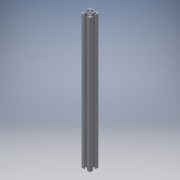
# Autodesk Inventor part: 20-2020_300mm
Saved by Autodesk Inventor 2019.4 (Build 234330000, 330)
## iProperties
Created: 2014-04-23
Part Number: 20-2020_300mm
Material: Aluminum 6105 T-5
Document SubType Name: Modeling
Designer: Ross Bowman
Density: 2.71 g/cm^3
Engineer: Ross Bowman
Catalog Web Link: 8020.net
Vendor: 80/20 Inc.
Mass: 43.1913 g
Surface Area: 184.633 cm^2
Volume: 15.9377 cm^3
Appearance: Aluminum - Flat
Company: 80/20 Inc.
Material: 6105-T5 Aluminum
Author: Ross Bowman
Keywords: 80/20 , 8020 , T-Slot , Extrusion
Autodesk Inventor part; units mm, degrees
ref_plane "YZ Plane" through (0, 0, 0) normal (1, 0, 0) x (0, 1, 0)
ref_plane "XZ Plane" through (0, 0, 0) normal (0, 1, 0) x (-1, 0, 0)
ref_plane "XY Plane" through (0, 0, 0) normal (0, 0, 1) x (1, 0, 0)
sketch "Sketch1" plane through (0, 0, 0) normal (0, 0, 1) x (1, 0, 0)
  arc A0 (-2.1249, -2.3045) -> (-0.804, -1.9351) centre (-1.5684, -1.748) ccw
  line L0 (-2.3045, -2.1249) -> (-2.1249, -2.3045)
  arc A1 (-1.9351, -0.804) -> (-2.3045, -2.1249) centre (-1.748, -1.5684) ccw
  arc A2 (-1.9351, 0.804) -> (-1.9351, -0.804) centre (0, 0) ccw
  arc A3 (-2.3045, 2.1249) -> (-1.9351, 0.804) centre (-1.748, 1.5684) ccw
  line L1 (-2.1249, 2.3045) -> (-2.3045, 2.1249)
  arc A4 (-0.804, 1.9351) -> (-2.1249, 2.3045) centre (-1.5684, 1.748) ccw
  arc A5 (0.804, 1.9351) -> (-0.804, 1.9351) centre (0, 0) ccw
  arc A6 (2.1249, 2.3045) -> (0.804, 1.9351) centre (1.5684, 1.748) ccw
  line L2 (2.3045, 2.1249) -> (2.1249, 2.3045)
  arc A7 (1.9351, 0.804) -> (2.3045, 2.1249) centre (1.748, 1.5684) ccw
  arc A8 (1.9351, -0.804) -> (1.9351, 0.804) centre (0, 0) ccw
  arc A9 (2.3045, -2.1249) -> (1.9351, -0.804) centre (1.748, -1.5684) ccw
  line L3 (2.1249, -2.3045) -> (2.3045, -2.1249)
  arc A10 (0.804, -1.9351) -> (2.1249, -2.3045) centre (1.5684, -1.748) ccw
  arc A11 (-0.804, -1.9351) -> (0.804, -1.9351) centre (0, 0) ccw
  arc A12 (9.492, 2.63) -> (10, 3.138) centre (9.492, 3.138) ccw
  line L4 (10, 3.138) -> (10, 8.5)
  arc A13 (10, 8.5) -> (8.5, 10) centre (8.5, 8.5) ccw
  line L5 (8.5, 10) -> (3.138, 10)
  arc A14 (3.138, 10) -> (2.63, 9.492) centre (3.138, 9.492) ccw
  line L6 (2.63, 9.492) -> (2.63, 9.008)
  arc A15 (2.63, 9.008) -> (3.138, 8.5) centre (3.138, 9.008) ccw
  line L7 (3.138, 8.5) -> (5.487, 8.5)
  arc A16 (5.995, 7.992) -> (5.487, 8.5) centre (5.487, 7.992) ccw
  line L8 (5.995, 7.992) -> (5.995, 7.2661)
  arc A17 (5.8462, 6.9069) -> (5.995, 7.2661) centre (5.487, 7.2661) ccw
  line L9 (5.8462, 6.9069) -> (2.7431, 3.8038)
  arc A18 (2.3839, 3.655) -> (2.7431, 3.8038) centre (2.3839, 4.163) ccw
  line L10 (2.3839, 3.655) -> (-2.3839, 3.655)
  arc A19 (-2.7431, 3.8038) -> (-2.3839, 3.655) centre (-2.3839, 4.163) ccw
  line L11 (-2.7431, 3.8038) -> (-5.8462, 6.9069)
  arc A20 (-5.995, 7.2661) -> (-5.8462, 6.9069) centre (-5.487, 7.2661) ccw
  line L12 (-5.995, 7.2661) -> (-5.995, 7.992)
  arc A21 (-5.487, 8.5) -> (-5.995, 7.992) centre (-5.487, 7.992) ccw
  line L13 (-5.487, 8.5) -> (-3.138, 8.5)
  arc A22 (-3.138, 8.5) -> (-2.63, 9.008) centre (-3.138, 9.008) ccw
  line L14 (-2.63, 9.008) -> (-2.63, 9.492)
  arc A23 (-2.63, 9.492) -> (-3.138, 10) centre (-3.138, 9.492) ccw
  line L15 (-3.138, 10) -> (-8.5, 10)
  arc A24 (-8.5, 10) -> (-10, 8.5) centre (-8.5, 8.5) ccw
  line L16 (-10, 8.5) -> (-10, 3.138)
  arc A25 (-10, 3.138) -> (-9.492, 2.63) centre (-9.492, 3.138) ccw
  line L17 (-9.492, 2.63) -> (-9.008, 2.63)
  arc A26 (-9.008, 2.63) -> (-8.5, 3.138) centre (-9.008, 3.138) ccw
  line L18 (-8.5, 3.138) -> (-8.5, 5.487)
  arc A27 (-7.992, 5.995) -> (-8.5, 5.487) centre (-7.992, 5.487) ccw
  line L19 (-7.992, 5.995) -> (-7.2661, 5.995)
  arc A28 (-6.9069, 5.8462) -> (-7.2661, 5.995) centre (-7.2661, 5.487) ccw
  line L20 (-6.9069, 5.8462) -> (-3.8038, 2.7431)
  arc A29 (-3.655, 2.3839) -> (-3.8038, 2.7431) centre (-4.163, 2.3839) ccw
  line L21 (-3.655, 2.3839) -> (-3.655, -2.3839)
  arc A30 (-3.8038, -2.7431) -> (-3.655, -2.3839) centre (-4.163, -2.3839) ccw
  line L22 (-3.8038, -2.7431) -> (-6.9069, -5.8462)
  arc A31 (-7.2661, -5.995) -> (-6.9069, -5.8462) centre (-7.2661, -5.487) ccw
  line L23 (-7.2661, -5.995) -> (-7.992, -5.995)
  arc A32 (-8.5, -5.487) -> (-7.992, -5.995) centre (-7.992, -5.487) ccw
  line L24 (-8.5, -5.487) -> (-8.5, -3.138)
  arc A33 (-8.5, -3.138) -> (-9.008, -2.63) centre (-9.008, -3.138) ccw
  line L25 (-9.008, -2.63) -> (-9.492, -2.63)
  arc A34 (-9.492, -2.63) -> (-10, -3.138) centre (-9.492, -3.138) ccw
  line L26 (-10, -3.138) -> (-10, -8.5)
  arc A35 (-10, -8.5) -> (-8.5, -10) centre (-8.5, -8.5) ccw
  line L27 (-8.5, -10) -> (-3.138, -10)
  arc A36 (-3.138, -10) -> (-2.63, -9.492) centre (-3.138, -9.492) ccw
  line L28 (-2.63, -9.492) -> (-2.63, -9.008)
  arc A37 (-2.63, -9.008) -> (-3.138, -8.5) centre (-3.138, -9.008) ccw
  line L29 (-3.138, -8.5) -> (-5.487, -8.5)
  arc A38 (-5.995, -7.992) -> (-5.487, -8.5) centre (-5.487, -7.992) ccw
  line L30 (-5.995, -7.992) -> (-5.995, -7.2661)
  arc A39 (-5.8462, -6.9069) -> (-5.995, -7.2661) centre (-5.487, -7.2661) ccw
  line L31 (-5.8462, -6.9069) -> (-2.7431, -3.8038)
  arc A40 (-2.3839, -3.655) -> (-2.7431, -3.8038) centre (-2.3839, -4.163) ccw
  line L32 (-2.3839, -3.655) -> (2.3839, -3.655)
  arc A41 (2.7431, -3.8038) -> (2.3839, -3.655) centre (2.3839, -4.163) ccw
  line L33 (2.7431, -3.8038) -> (5.8462, -6.9069)
  arc A42 (5.995, -7.2661) -> (5.8462, -6.9069) centre (5.487, -7.2661) ccw
  line L34 (5.995, -7.2661) -> (5.995, -7.992)
  arc A43 (5.487, -8.5) -> (5.995, -7.992) centre (5.487, -7.992) ccw
  line L35 (5.487, -8.5) -> (3.138, -8.5)
  arc A44 (3.138, -8.5) -> (2.63, -9.008) centre (3.138, -9.008) ccw
  line L36 (2.63, -9.008) -> (2.63, -9.492)
  arc A45 (2.63, -9.492) -> (3.138, -10) centre (3.138, -9.492) ccw
  line L37 (3.138, -10) -> (8.5, -10)
  arc A46 (8.5, -10) -> (10, -8.5) centre (8.5, -8.5) ccw
  line L38 (10, -8.5) -> (10, -3.138)
  arc A47 (10, -3.138) -> (9.492, -2.63) centre (9.492, -3.138) ccw
  line L39 (9.492, -2.63) -> (9.008, -2.63)
  arc A48 (9.008, -2.63) -> (8.5, -3.138) centre (9.008, -3.138) ccw
  line L40 (8.5, -3.138) -> (8.5, -5.487)
  arc A49 (7.992, -5.995) -> (8.5, -5.487) centre (7.992, -5.487) ccw
  line L41 (7.992, -5.995) -> (7.2661, -5.995)
  arc A50 (6.9069, -5.8462) -> (7.2661, -5.995) centre (7.2661, -5.487) ccw
  line L42 (6.9069, -5.8462) -> (3.8038, -2.7431)
  arc A51 (3.655, -2.3839) -> (3.8038, -2.7431) centre (4.163, -2.3839) ccw
  line L43 (3.655, -2.3839) -> (3.655, 2.3839)
  arc A52 (3.8038, 2.7431) -> (3.655, 2.3839) centre (4.163, 2.3839) ccw
  line L44 (3.8038, 2.7431) -> (6.9069, 5.8462)
  arc A53 (7.2661, 5.995) -> (6.9069, 5.8462) centre (7.2661, 5.487) ccw
  line L45 (7.2661, 5.995) -> (7.992, 5.995)
  arc A54 (8.5, 5.487) -> (7.992, 5.995) centre (7.992, 5.487) ccw
  line L46 (8.5, 5.487) -> (8.5, 3.138)
  arc A55 (8.5, 3.138) -> (9.008, 2.63) centre (9.008, 3.138) ccw
  line L47 (9.008, 2.63) -> (9.492, 2.63)
  constraints: 112 point on circle, 96 end point, 56 centre point
extrude "Extrusion1" add sketch "Sketch1" against normal blind 100
move faces "Move1" translate (0, 0, 200) faces at (-7.4957, -7.9957, 0)
body "Solid1"
